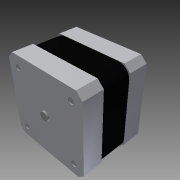
# Autodesk Inventor part: NEMA17
Saved by Autodesk Inventor 2014 (Build 180170000, 170)
## iProperties
Created: 2013-12-12
Part Number: NEMA17
Material: Generic
Document SubType Name: Modeling
Designer: Bram
Density: 1 g/cm^3
Appearance: Default
Author: Bram
Autodesk Inventor part; units mm, degrees
ref_plane "YZ Plane" through (0, 0, 0) normal (1, 0, 0) x (0, 1, 0)
ref_plane "XZ Plane" through (0, 0, 0) normal (0, 1, 0) x (-1, 0, 0)
sketch "Sketch1" plane through (0, 0, 0) normal (0, 1, 0) x (-1, 0, 0)
  line L0 (0, 0) -> (-42.3, 0)
  line L1 (-42.3, 0) -> (-42.3, 42.3)
  line L2 (-42.3, 42.3) -> (0, 42.3)
  line L3 (0, 42.3) -> (0, 0)
  dimension "d0" = 42.3
  dimension "d1" = 42.3
  constraints: 8 end point, 2 parallel, 1 horizontal, 1 perpendicular
  measures "d0" distance of L1.end L2.end
  measures "d1" distance of L0.end L1.end
extrude "Extrusion1" add sketch "Sketch1" along normal blind 10
chamfer "Chamfer1" distance 3 angle 45 4 edges at (42.3, 5, 42.3) (0, 5, 42.3) (0, 5, 0) (42.3, 5, 0)
sketch "Sketch2" plane through (0, 10, 0) normal (0, 1, 0) x (1, 0, 0)
  line L0 (0.15, -42.15) -> (42.15, -42.15)
  line L1 (42.15, -42.15) -> (42.15, -0.15)
  line L2 (42.15, -0.15) -> (0.15, -0.15)
  line L3 (0.15, -0.15) -> (0.15, -42.15)
  line L4 (0.15, -42.15) -> (42.15, -0.15) construction
  line L5 (42.15, -42.15) -> (0.15, -0.15) construction
  point P0 (0, 0)
  point P1 (21.15, -21.15)
  dimension "d7" = 42
  dimension "d8" = 42
  constraints: 12 end point, 2 midpoint, 2 parallel, 1 horizontal, 1 perpendicular
  measures "d7" distance of L2.end L1.end
  measures "d8" distance of L1.end L0.end
extrude "Extrusion2" add sketch "Sketch2" along normal blind 14
fillet "Fillet1" radius 6 4 edges at (42.15, 17, 42.15) (42.15, 17, 0.15) (0.15, 17, 42.15) (0.15, 17, 0.15)
sketch "Sketch3" plane through (0, 24, 0) normal (0, 1, 0) x (1, 0, 0)
  line L0 (0, -42.3) -> (42.3, -42.3)
  line L1 (42.3, -42.3) -> (42.3, 0)
  line L2 (42.3, 0) -> (0, 0)
  line L3 (0, 0) -> (0, -42.3)
  line L4 (0, -42.3) -> (42.3, 0) construction
  line L5 (42.3, -42.3) -> (0, 0) construction
  point P0 (0, 0)
  point P1 (21.15, -21.15)
  dimension "d12" = 42.3
  dimension "d13" = 42.3
  constraints: 12 end point, 2 midpoint, 2 parallel, 1 horizontal, 1 perpendicular
  measures "d12" distance of L2.end L1.end
  measures "d13" distance of L1.end L0.end
extrude "Extrusion3" add sketch "Sketch3" along normal blind 10
chamfer "Chamfer2" distance 3 angle 45 4 edges at (42.3, 29, 42.3) (42.3, 29, 0) (0, 29, 0) (0, 29, 42.3)
ref_plane "Work Plane1" through (39.3, 0, 21.15) normal (0, 0, -1) x (-1, 0, 0)
sketch "Sketch4" plane through (0, 34, 0) normal (0, 1, 0) x (1, 0, 0)
  circle A0 centre (21.15, -21.15) radius 11
  point P0 (0, 0)
  dimension "d19" = 22
  constraints: 1 centre point
  measures "d19" diameter of A0
extrude "Extrusion4" add sketch "Sketch4" along normal blind 2.03
sketch "Sketch5" plane through (21.15, 36.03, 21.15) normal (0, 1, 0) x (1, 0, 0)
  circle A0 centre (0, 0) radius 11 projected
  circle A1 centre (0, 0) radius 2.26
  point P0 (-21.15, 21.15)
  dimension "d22" = 4.52
  constraints: 1 centre point, 1 coincident
  measures "d22" diameter of A1
extrude "Extrusion5" add sketch "Sketch5" along normal blind 14 contours A1
sketch "Sketch6" plane through (0, 34, 0) normal (0, 1, 0) x (1, 0, 0)
  circle A0 centre (21.15, -21.15) radius 11 projected
  line L0 (5.655, -36.645) -> (36.645, -5.655) construction
  line L1 (36.645, -36.645) -> (5.655, -5.655) construction
  circle A1 centre (5.655, -5.655) radius 1.5
  circle A2 centre (36.645, -5.655) radius 1.5
  circle A3 centre (36.645, -36.645) radius 1.5
  circle A4 centre (5.655, -36.645) radius 1.5
  point P0 (0, 0)
  dimension "d25" = 30.99
  dimension "d26" = 30.99
  dimension "d27" = 3
  dimension "d28" = 3
  dimension "d29" = 3
  dimension "d30" = 3
  constraints: 4 centre point, 4 coincident, 4 end point, 2 midpoint
  measures "d25" distance of L1.end L0.end
  measures "d26" distance of L0.end L1.start
  measures "d27" diameter of A1
  measures "d28" diameter of A2
  measures "d29" diameter of A3
  measures "d30" diameter of A4
extrude "Extrusion6" cut sketch "Sketch6" against normal blind 4.5 contours A1 | A2 | A3 | A4
thread "Thread1" size "M3x0.5" class "6H" standard "ANSI Metric M Profile" full length
thread "Thread2" size "M3x0.5" class "6H" standard "ANSI Metric M Profile" full length
thread "Thread3" size "M3x0.5" class "6H" standard "ANSI Metric M Profile" full length
thread "Thread4" size "M3x0.5" class "6H" standard "ANSI Metric M Profile" full length
sketch "Sketch7" plane through (0, 0, 0) normal (0, -1, 0) x (1, 0, 0)
  circle A0 centre (21.15, 21.15) radius 2.25
  point P0 (0, 0)
  dimension "d41" = 4.5
  constraints: 1 centre point
  measures "d41" diameter of A0
extrude "Extrusion7" add sketch "Sketch7" along normal blind 1
sketch "Sketch8" plane through (0, 0, 0) normal (0, -1, 0) x (1, 0, 0)
  line L0 (5.65, 5.65) -> (36.65, 36.65) construction
  line L1 (36.65, 5.65) -> (5.65, 36.65) construction
  circle A0 centre (5.65, 36.65) radius 1.5
  circle A1 centre (36.65, 36.65) radius 1.5
  circle A2 centre (36.65, 5.65) radius 1.5
  circle A3 centre (5.65, 5.65) radius 1.5
  point P0 (0, 0)
  point P1 (21.15, 21.15)
  dimension "d44" = 31
  dimension "d45" = 31
  dimension "d46" = 3
  dimension "d47" = 3
  dimension "d48" = 3
  dimension "d49" = 3
  constraints: 4 centre point, 4 coincident, 4 end point, 2 midpoint
  measures "d44" distance of L1.end L0.end
  measures "d45" distance of L0.end L1.start
  measures "d46" diameter of A0
  measures "d47" diameter of A1
  measures "d48" diameter of A2
  measures "d49" diameter of A3
extrude "Extrusion8" cut sketch "Sketch8" against normal blind 0.5
body "Solid1"
